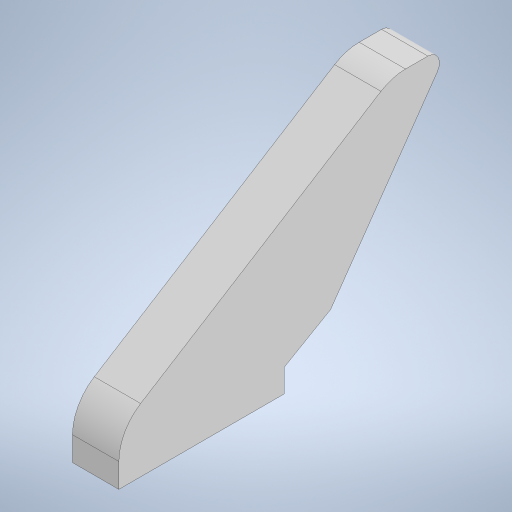
# Autodesk Inventor part: vertical_tail
Saved by Autodesk Inventor 2024 (Build 280153000, 153)
## iProperties
Created: 2023-06-07
Part Number: vertical_tail
Material: Generic
Document SubType Name: Modeling
Designer: tamiz
Density: 1 g/cm^3
Appearance: Default
Author: tamiz
Autodesk Inventor part; units mm, degrees
ref_plane "YZ Plane" through (0, 0, 0) normal (1, 0, 0) x (0, 1, 0)
ref_plane "XZ Plane" through (0, 0, 0) normal (0, 1, 0) x (-1, 0, 0)
ref_plane "XY Plane" through (0, 0, 0) normal (0, 0, 1) x (1, 0, 0)
sketch "Sketch18" plane through (0, 0, 0) normal (1, 0, 0) x (0, 1, 0)
  line L0 (3086.1, 2980.944) -> (3721.5332, 2980.944)
  line L1 (3086.1, 2980.944) -> (3086.1, -1371.6)
  line L2 (3086.1, -1371.6) -> (3695.7, -1371.6)
  line L3 (3695.7, -1371.6) -> (4397.2643, -2586.7449)
  line L4 (4397.2643, -2586.7449) -> (3787.6643, -1530.8868)
  line L5 (4397.2643, -2586.7449) -> (8411.8339, -5397.7769)
  line L6 (4397.2643, -2586.7449) -> (9298.1489, -2586.7449) construction
  line L7 (8891.46, -5148.0993) -> (8891.46, -4559.283)
  line L8 (8706.1333, -3913.0983) -> (4755.4065, 2407.9287)
  arc A0 (4755.4065, 2407.9287) -> (3721.5332, 2980.944) centre (3721.5332, 1761.744) ccw
  arc A1 (8891.46, -4559.283) -> (8706.1333, -3913.0983) centre (7672.26, -4559.283) ccw
  arc A2 (8411.8339, -5397.7769) -> (8891.46, -5148.0993) centre (8586.66, -5148.0993) ccw
  point P0 (0, 0)
  point P1 (8891.46, -5733.6147)
  point P2 (8891.46, -4209.6147)
  dimension "d85" = 4352.544
  dimension "d89" = 5486.4
  dimension "d90" = 35
  dimension "d91" = 1524
  dimension "d92" = 1219.2
  dimension "d93" = 304.8
  constraints: 18 end point, 6 point on circle, 6 tangent, 5 point on line, 3 centre point, 2 vertical, 1 equal length, 1 equal radius, 1 horizontal, 1 perpendicular
  measures "d85" distance of L0.start L1.end
  measures "d89" distance of L3.end point (8891.46, -5733.615)
  measures "d90" angle of L5 L6
  measures "d91" distance of point (8891.46, -5733.615) point (8891.46, -4209.615)
  measures "d92" radius of A0
  measures "d93" radius of A2
extrude "Extrusion16" add sketch "Sketch18" along normal mid plane 1219.2
body "Solid2"
